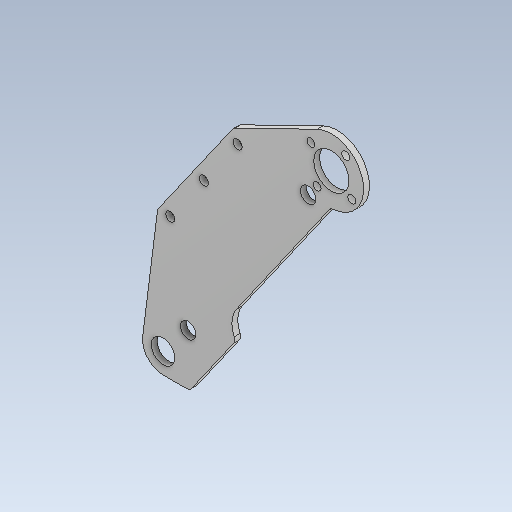
# Autodesk Inventor part: FrontLink_frame
Saved by Autodesk Inventor 2020 (Build 240168000, 168)
## iProperties
Created: 2021-10-03
Part Number: FrontLink_frame
Material: GFRP
Document SubType Name: Modeling
Designer: Masato Kubotera
Density: 1.75 g/cm^3
Appearance: 滑らか - 淡い灰色
Description: GFRP T2
Author: Masato Kubotera
Autodesk Inventor part; units mm, degrees
ref_plane "YZ Plane" through (0, 0, 0) normal (1, 0, 0) x (0, 1, 0)
ref_plane "XZ Plane" through (0, 0, 0) normal (0, 1, 0) x (-1, 0, 0)
ref_plane "XY Plane" through (0, 0, 0) normal (0, 0, 1) x (1, 0, 0)
derived "Link_basis.ipt"
sketch "スケッチ1" plane through (0, 0, 0) normal (0, 0, 1) x (1, 0, 0)
  circle A0 centre (0, 0) radius 6
  circle A1 centre (-57.3576, -81.9152) radius 4
  arc A2 (-64.3015, -81.0305) -> (-57.3576, -88.9152) centre (-57.3576, -81.9152) ccw
  arc A3 (-0.1434, -10.9991) -> (-4.8354, 9.8802) centre (0, 0) ccw
  line L0 (-58.3761, -41.5269) -> (-32.5651, -4.6651) construction
  line L1 (-32.5651, -4.6651) -> (-28.4694, -7.533) construction
  line L2 (-28.4694, -7.533) -> (-54.2803, -44.3948) construction
  line L3 (-54.2803, -44.3948) -> (-58.3761, -41.5269) construction
  line L4 (-58.3761, -41.5269) -> (-28.4694, -7.533) construction
  line L5 (-32.5651, -4.6651) -> (-54.2803, -44.3948) construction
  line L6 (-56.3282, -42.9609) -> (-30.5172, -6.099) construction
  circle A4 centre (-54.8942, -40.913) radius 1.55
  circle A5 centre (-43.4227, -24.5299) radius 1.55
  line L7 (-45.4706, -23.096) -> (-41.3748, -25.9639) construction
  circle A6 centre (-31.9512, -8.1469) radius 1.55
  line L8 (-59.1952, -40.9534) -> (-33.3843, -4.0915)
  line L9 (-33.3843, -4.0915) -> (-4.8354, 9.8802)
  line L10 (-59.1952, -40.9534) -> (-64.3015, -81.0305)
  line L11 (-32.3614, -57.0111) -> (-0.1434, -10.9991)
  line L12 (0, 0) -> (32, 0) construction
  line L13 (32, 0) -> (32, 20) construction
  circle A7 centre (32, 20) radius 4
  arc A8 (38.9218, 15.1533) -> (32, 28.45) centre (32, 20) ccw
  line L14 (32, 20) -> (32, 37) construction
  circle A9 centre (32, 37) radius 4 construction
  circle A10 centre (32, 37) radius 8.45 construction
  line L15 (-57.3576, -81.9152) -> (0, 0) construction
  circle A11 centre (0, 0) radius 8.5 construction
  line L16 (0, 0) -> (4.8754, 6.9628) construction
  circle A12 centre (4.8754, 6.9628) radius 1.35
  circle A13 centre (32, 20) radius 7 construction
  arc A14 (-64.3015, -81.0305) -> (-53.3426, -76.1811) centre (-57.3576, -81.9152) ccw construction
  line L17 (-51.6236, -85.9302) -> (-33.7808, -60.4482)
  line L18 (38.9218, 15.1533) -> (-18.4358, -66.7619)
  line L19 (32, 20) -> (-25.3576, -61.9152) construction
  circle A15 centre (-25.3576, -61.9152) radius 4
  circle A16 centre (-25.3576, -61.9152) radius 8 construction
  arc A17 (-0.0917, -11.0996) -> (11.1, 0) centre (0, 0) ccw
  line L20 (25.0782, 24.8467) -> (10.3989, 3.8825)
  line L21 (-0.0917, -11.0996) -> (-32.2795, -57.0685)
  arc A18 (-32.2795, -57.0685) -> (-18.4358, -66.7619) centre (-25.3576, -61.9152) ccw
  arc A19 (-32.3614, -57.0111) -> (-32.5799, -66.4914) centre (-25.3576, -61.9152) ccw
  line L22 (-6.9628, 4.8754) -> (0, 0) construction
  circle A20 centre (-6.9628, 4.8754) radius 1.35
  circle A21 centre (-4.8754, -6.9628) radius 1.35
  circle A22 centre (6.9628, -4.8754) radius 1.35
  line L23 (-6.1434, -38.7459) -> (8.196, -18.2671) construction
  line L24 (8.196, -18.2671) -> (12.2917, -21.135) construction
  line L25 (12.2917, -21.135) -> (-2.0477, -41.6138) construction
  line L26 (-2.0477, -41.6138) -> (-6.1434, -38.7459) construction
  line L27 (-6.1434, -38.7459) -> (12.2917, -21.135) construction
  line L28 (8.196, -18.2671) -> (-2.0477, -41.6138) construction
  line L29 (10.2439, -19.701) -> (-4.0955, -40.1798) construction
  line L30 (1.0263, -28.5065) -> (5.122, -31.3744) construction
  circle A23 centre (8.8099, -21.7489) radius 1.55
  circle A24 centre (-2.6616, -38.132) radius 1.55
  line L31 (7.185, 8.4608) -> (11.1, 14.052)
  line L32 (32, 28.45) -> (21.1816, 28.45)
  arc A25 (32, 28.45) -> (25.0782, 24.8467) centre (32, 20) ccw construction
  line L33 (-32.5799, -66.4914) -> (-48.2812, -88.9152)
  line L34 (-57.3576, -88.9152) -> (-48.2812, -88.9152)
  arc A26 (-57.3576, -88.9152) -> (-51.6236, -85.9302) centre (-57.3576, -81.9152) ccw construction
  line L35 (12.7716, -28.3397) -> (-7.9116, -10.9844) construction
  line L36 (-7.9116, -10.9844) -> (9.4437, 9.6988) construction
  line L37 (9.4437, 9.6988) -> (30.1269, -7.6565) construction
  line L38 (30.1269, -7.6565) -> (12.7716, -28.3397) construction
  line L39 (12.7716, -28.3397) -> (9.4437, 9.6988) construction
  line L40 (-7.9116, -10.9844) -> (30.1269, -7.6565) construction
  line L41 (0.766, -0.6428) -> (21.4492, -17.9981) construction
  circle A27 centre (-7.9116, -10.9844) radius 2.639
  circle A28 centre (-4.8754, -6.9628) radius 2.4 construction
  line L42 (-42.1647, -109.0339) -> (-64.2818, -93.5473) construction
  line L43 (-64.2818, -93.5473) -> (-48.7952, -71.4302) construction
  line L44 (-48.7952, -71.4302) -> (-26.6781, -86.9168) construction
  line L45 (-26.6781, -86.9168) -> (-42.1647, -109.0339) construction
  line L46 (-42.1647, -109.0339) -> (-48.7952, -71.4302) construction
  line L47 (-64.2818, -93.5473) -> (-26.6781, -86.9168) construction
  line L48 (-56.5385, -82.4888) -> (-34.4214, -97.9753) construction
  circle A29 centre (-48.7952, -71.4302) radius 2.639
  line L49 (11.1, 0) -> (11.1, 14.052)
  line L50 (11.1, 14.052) -> (21.1816, 28.45)
  arc A30 (11.1, 0) -> (7.185, 8.4608) centre (0, 0) ccw construction
  point P0 (3.0742, -29.9404)
  point P1 (11.1076, -9.3204)
  point P2 (-45.4799, -90.2321)
  dimension "d5" = 27
  dimension "d6" = 27
  dimension "d9" = 5
  dimension "d12" = 4.8
  dimension "d13" = 27
  dimension "d14" = 27
  dimension "d17" = 0
  dimension "d18" = 1
  dimension "d19" = 1
  dimension "d20" = 5.278
  dimension "d21" = 5.278
  measures "d5" distance of L36.end L37.end
  measures "d6" distance of L35.end L36.end
  measures "d9" angle of L36 L15
  measures "d12" diameter of A28
  measures "d13" distance of L43.end L44.end
  measures "d14" distance of L42.end L43.end
  measures "d17" angle of L15 L43
  measures "d18" distance from line of point (0, 0) L36
  measures "d19" distance from line of A1.centre L43
  measures "d20" diameter of A27
  measures "d21" diameter of A29
extrude "押し出し1" add sketch "スケッチ1" along normal blind 2 contours L10 L8 L9 A3 L11 A19 L33 L34 A2
fillet "フィレット1" radius 2 3 edges at (-33.3843, -4.0915, 1) (-59.1952, -40.9534, 1) (-0.1434, -10.9991, 1)
fillet "フィレット2" radius 2 2 edges at (-32.5799, -66.4914, 1) (-48.2812, -88.9152, 1)
equation "\"d21\" = d20"
